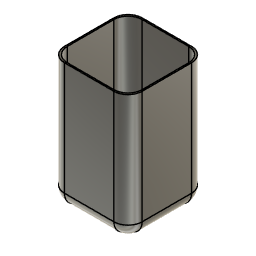
couvre_micro_elgato v2 (Autodesk Fusion 360 design; units mm, degrees)
Autodesk Fusion 360 part; units mm, degrees
note: some values were not read from the file. Set by a fixed rule: which sketch regions a step uses.
sketch "Esquisse1" plane through (0, 0, 0) normal (0, 0, 1) x (1, 0, 0)
  line L0 (0, 0) -> (53, 0)
  line L1 (53, 0) -> (53, 53)
  line L2 (53, 53) -> (0, 53)
  line L3 (0, 53) -> (0, 0)
  line L4 (54, -1) -> (54, 54)
  line L5 (54, 54) -> (-1, 54)
  line L6 (-1, 54) -> (-1, -1)
  line L7 (-1, -1) -> (54, -1)
  line L8 (26.5, 53) -> (26.5, 0)
  circle A0 centre (26.5, 26.5) radius 5
  dimension "d4" = 53
  dimension "d5" = 53
  dimension "d6" = 1
  dimension "d20" = 10
  constraint horizontal L0
  constraint vertical L1
  constraint horizontal L2
  constraint vertical L3
  constraint coincident L0.start L3.end
  constraint midpoint L2 L8.start
  constraint midpoint L0 L8.end
  constraint midpoint L8 A0.centre
  measures "d4" distance of L0.start L0.end
  measures "d5" distance of L0.start L2.end
  measures "d20" diameter of A0
extrude "Extrusion1" add sketch "Esquisse1" along normal blind 90
extrude "Extrusion2" add sketch "Esquisse1" along normal blind 1 contours L0 L2 L3 L8 A0 | L0 L1 L2 L8 A0 | L8 A0 | L8 A0
fillet "Congé1" radius 10 4 edges at (0, 53, 45.5) (53, 53, 45.5) (53, 0, 45.5) (0, 0, 45.5)
fillet "Congé2" radius 10 8 edges at (50.0711, 50.0711, 1) (53, 26.5, 1) (50.0711, 2.9289, 1) (26.5, 0, 1) (2.9289, 2.9289, 1) (0, 26.5, 1) (2.9289, 50.0711, 1) (26.5, 53, 1)
fillet "Congé3" radius 10 4 edges at (-1, 54, 45) (54, 54, 45) (54, -1, 45) (-1, -1, 45)
fillet "Congé4" radius 10 8 edges at (54, 26.5, 0) (51.0711, 51.0711, 0) (26.5, 54, 0) (1.9289, 51.0711, 0) (-1, 26.5, 0) (1.9289, 1.9289, 0) (26.5, -1, 0) (51.0711, 1.9289, 0)
extrude "Extrusion3" cut sketch "Esquisse1" along normal blind 1 contours L8 A0 | L8 A0
equation "base_largeur = 53 mm"
equation "epaisseur = 1 mm"
equation "hauteur = 90 mm"
equation "d4 = base_largeur"
equation "d5 = base_largeur"
equation "d6 = epaisseur"
equation "d7 = hauteur"
equation "d9 = epaisseur"
equation "angle_int = 10 mm"
equation "d13 = angle_int"
equation "d15 = angle_int"
equation "d17 = angle_int"
equation "d19 = angle_int"
equation "d21 = epaisseur"
